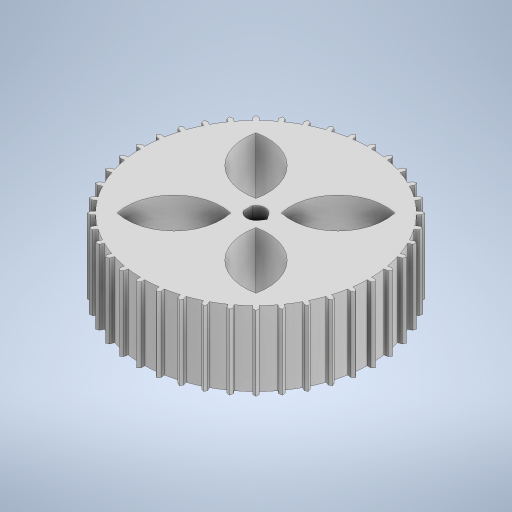
# Autodesk Inventor part: flower_wheel_rev1
Saved by Autodesk Inventor 2024 (Build 280153000, 153)
## iProperties
Created: 2023-11-25
Part Number: flower_wheel_rev1
Material: Generic
Document SubType Name: Modeling
Designer: jerem
Density: 1 g/cm^3
Appearance: Default
Author: jerem
## iProperties of the stored document WHEEL_SPIKEY_3DPrint.ipt
Created: 2023-11-27
Part Number: WHEEL_SPIKEY_3DPrint
Material: Generic
Document SubType Name: Modeling
Designer: jerem
Density: 1 g/cm^3
Appearance: Default
Author: jerem
Autodesk Inventor part; units mm, degrees
ref_plane "YZ Plane" through (0, 0, 0) normal (1, 0, 0) x (0, 1, 0)
ref_plane "XZ Plane" through (0, 0, 0) normal (0, 1, 0) x (-1, 0, 0)
sketch "Sketch1" plane through (0, 0, 0) normal (0, 1, 0) x (-1, 0, 0)
  circle A0 centre (0, 0) radius 38.1
  arc A1 (2.75, 1.4309) -> (2.75, -1.4309) centre (0, 0) ccw
  line L0 (-2.5627, -1.7443) -> (-3.75, 0)
  line L1 (-3.75, 0) -> (0, 0)
  line L2 (-3.75, 0) -> (-2.5627, 1.7443)
  line L3 (2.75, 1.4309) -> (2.75, -1.4309)
  point P0 (-3.1, 0)
  dimension "d0" = 76.2
  dimension "d1" = 6.2
  dimension "d116" = 3.75
  dimension "d117" = 2.75
  constraints: 8 end point, 4 point on circle, 2 centre point, 2 coincident, 2 tangent, 1 horizontal, 1 vertical
  measures "d0" diameter of A0
  measures "d1" diameter of A1
  measures "d116" distance of L0.end L1.end
  measures "d117" distance from line of L3 point (0, 0)
extrude "Extrusion1" add sketch "Sketch1" along normal blind 25
ref_plane "Work Plane1" through (-38.1, 0, 0) normal (1, 0, 0) x (0, 0, -1)
sketch "Sketch4" plane through (0, 25, 0) normal (0, 1, 0) x (1, 0, 0)
  circle A0 centre (0, 0) radius 38.1 projected
  line L0 (-38.1, 0) -> (-40.1, 0)
  line L1 (-40.1, 0) -> (-40.1, 0)
  line L2 (-39.35, -0.75) -> (-38.0926, -0.75)
  line L3 (-40.1, 0) -> (-40.1, 0)
  line L4 (-39.35, 0.75) -> (-38.0926, 0.75)
  circle A1 centre (0, 0) radius 38.1
  line L5 (-40.1, 0) -> (-39.35, 0.75)
  line L6 (-40.1, 0) -> (-39.35, -0.75)
  point P0 (-40.1, -0.75)
  point P1 (-40.1, 0.75)
  dimension "d118" = 2
  dimension "d119" = 0.75
  dimension "d120" = 0.75
  dimension "d121" = 0.75
  dimension "d122" = 0.75
  dimension "d123" = 0.75
  constraints: 14 end point, 4 point on line, 2 perpendicular, 2 point on circle, 2 symmetric about line, 1 centre point, 1 coincident, 1 concentric, 1 horizontal
  measures "d118" distance of L0.start L0.end
  measures "d119" distance of L0.end point (-40.1, -0.75)
  measures "d120" distance of L3.end point (-40.1, 0.75)
  measures "d121" distance of L4.start point (-40.1, 0.75)
  measures "d122" distance of L1.end point (-40.1, -0.75)
  measures "d123" distance of L2.start point (-40.1, -0.75)
extrude "Extrusion4" add sketch "Sketch4" against normal blind 25 contours A0 L0 L5 L4 | L2 L6 L0 A0
pattern_circular "Circular Pattern4" count 40 over 360 about axis through (0, 0, 0) along (0, 1, 0) of "Extrusion4"
sketch "Sketch5" plane through (0, 0, 0) normal (0, -1, 0) x (1, 0, 0)
  circle A0 centre (0, 0) radius 6
  circle A1 centre (0, 0) radius 33
  line L0 (0, 0) -> (-23.3345, -23.3345)
  line L1 (0, 0) -> (33, 0) construction
  line L2 (0, 0) -> (-33, 0)
  line L3 (0, 0) -> (0, -33)
  line L4 (0, 0) -> (-23.3345, 23.3345)
  line L5 (0, 0) -> (23.3345, -23.3345)
  line L6 (0, 0) -> (23.3345, 23.3345)
  arc A2 (-4.2426, -4.2426) -> (-23.3345, -23.3345) centre (-7.7161, -19.8611) ccw
  arc A3 (-23.3345, 23.3345) -> (-4.2426, 4.2426) centre (-7.7161, 19.8611) ccw
  arc A4 (23.3345, -23.3345) -> (4.2426, -4.2426) centre (7.7161, -19.8611) ccw
  arc A5 (4.2426, 4.2426) -> (23.3345, 23.3345) centre (7.7161, 19.8611) ccw
  arc A6 (-4.2426, 4.2426) -> (-23.3345, 23.3345) centre (-19.8611, 7.7161) ccw
  arc A7 (23.3345, 23.3345) -> (4.2426, 4.2426) centre (19.8611, 7.7161) ccw
  arc A8 (4.2426, -4.2426) -> (23.3345, -23.3345) centre (19.8611, -7.7161) ccw
  arc A9 (-23.3345, -23.3345) -> (-4.2426, -4.2426) centre (-19.8611, -7.7161) ccw
  dimension "d129" = 12
  dimension "d131" = 135
  dimension "d132" = 16
  constraints: 19 point on circle, 14 end point, 13 symmetric about line, 9 centre point, 2 coincident, 2 horizontal, 1 equal length, 1 perpendicular, 1 point on line, 10 other
  measures "d131" angle of L0 L1
  measures "d132" radius of A2
extrude "Extrusion5" cut sketch "Sketch5" against normal through all contours A7 L6 | L6 A5 | A4 L5 | L5 A8 | A3 L4 | L4 A6 | A9 L0 | L0 A2
sketch "Sketch6" plane through (0, 0, 0) normal (0, -1, 0) x (1, 0, 0)
  circle A0 centre (0, 0) radius 36.0724
  constraints: 1 centre point, 1 coincident
extrude "Extrusion6" add sketch "Sketch6" against normal blind 2
body "Solid1"
